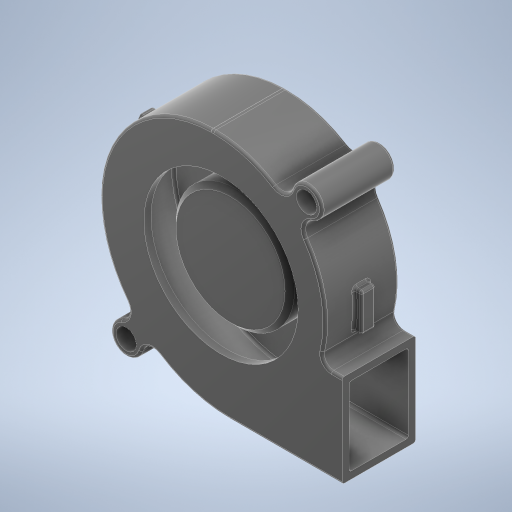
# Autodesk Inventor part: 5015 Fan
Saved by Autodesk Inventor 2024 (Build 280153000, 153)
## iProperties
Created: 2025-01-19
Part Number: 5015 Fan
Material: ABS Plastic
Document SubType Name: Modeling
Designer: Ishaan
Density: 1.06 g/cm^3
Appearance: Smooth - Black
Author: Ishaan
Autodesk Inventor part; units mm, degrees
ref_plane "YZ Plane" through (0, 0, 0) normal (1, 0, 0) x (0, 1, 0)
ref_plane "XZ Plane" through (0, 0, 0) normal (0, 1, 0) x (-1, 0, 0)
ref_plane "XY Plane" through (0, 0, 0) normal (0, 0, 1) x (1, 0, 0)
sketch "Sketch1" plane through (0, 0, 0) normal (0, 0, 1) x (1, 0, 0)
  line L0 (-51.0368, 43.6346) -> (74.9868, 43.6346) construction
  line L1 (74.9868, 43.6346) -> (74.9868, -48.5034) construction
  line L2 (74.9868, -48.5034) -> (-51.0368, -48.5034) construction
  line L3 (-51.0368, -48.5034) -> (-51.0368, 43.6346) construction
  circle A0 centre (0, 0) radius 16.25 construction
  line L4 (0, 0) -> (-20, 0) construction
  line L5 (-20, 0) -> (-20, -23.5) construction
  line L6 (-20, -23.5) -> (0, -23.5) construction
  line L7 (0, -23.5) -> (0, 0) construction
  line L8 (0, 0) -> (18, 0) construction
  line L9 (18, 0) -> (18, 20.5) construction
  line L10 (18, 20.5) -> (0, 20.5) construction
  line L11 (0, 20.5) -> (0, 0) construction
  circle A1 centre (-20, -23.5) radius 2.15 construction
  circle A2 centre (-20, -23.5) radius 3.25
  circle A3 centre (18, 20.5) radius 3.25
  line L12 (25.5, -27.3) -> (-25.5, -27.3)
  line L13 (-25.5, -27.3) -> (-25.5, 23.7)
  line L14 (-25.5, 23.7) -> (25.5, 23.7)
  line L15 (25.5, 23.7) -> (25.5, -27.3)
  line L16 (25.5, -27.3) -> (-25.5, 23.7) construction
  line L17 (-25.5, -27.3) -> (25.5, 23.7) construction
  line L18 (25.5, -7.8) -> (20.5964, -7.8)
  arc A4 (20.5964, -7.8) -> (-1.5, 23.7) centre (-1.5, 0.2) ccw
  arc A5 (-1.5, 23.7) -> (-25.5, 0) centre (-1.7981, 0) ccw
  arc A6 (-25.5, 0) -> (1.8, -27.3) centre (1.8, 0) ccw
  circle A7 centre (12.4829, 22.1198) radius 2.5
  circle A8 centre (19.8402, 15.0524) radius 2.5
  circle A9 centre (-21.8953, -18.0713) radius 2.5
  circle A10 centre (-14.4446, -24.9831) radius 2.5
  line L19 (-51.0368, 43.6346) -> (74.9868, 43.6346) construction
  line L20 (74.9868, 43.6346) -> (74.9868, -48.5034) construction
  line L21 (74.9868, -48.5034) -> (-51.0368, -48.5034) construction
  line L22 (-51.0368, -48.5034) -> (-51.0368, 43.6346) construction
  line L23 (25.5, -27.3) -> (25.5, -7.8)
  point P0 (0, -1.8)
  point P1 (-19.9074, -16.5553)
  point P2 (-21.0713, -20.4316)
  point P3 (-16.86, -24.3383)
  point P4 (-13.0818, -22.8872)
  point P5 (17.7883, 13.6243)
  point P6 (19.0401, 17.4209)
  point P7 (14.8816, 21.4156)
  point P8 (11.1384, 20.0122)
  point P9 (-2.0962, 23.7)
  point P10 (18.5679, 23.7)
  point P11 (17.4321, 23.7)
  point P12 (25.5, -17.55)
  dimension "d1" = 32.5
  dimension "d14" = 20
  dimension "d15" = 23.5
  dimension "d16" = 18
  dimension "d17" = 20.5
  dimension "d38" = 4.3
  dimension "d39" = 6.5
  dimension "d40" = 6.5
  dimension "d41" = 51
  dimension "d42" = 51
  dimension "d44" = 1.8
  dimension "d45" = 19.5
  dimension "d50" = 1.5
  dimension "d56" = 23.5
  dimension "d59" = 5
  dimension "d100" = 17.55
  constraints: 32 end point, 12 tangent, 11 centre point, 6 coincident, 6 parallel, 6 point on circle, 5 horizontal, 5 point on line, 4 perpendicular, 4 vertical, 3 equal radius, 3 midpoint, 1 horizontal alignment, 4 other
  measures "d1" diameter of A0
  measures "d14" distance of L6.end L5.end
  measures "d15" distance of L5.end L4.end
  measures "d16" distance of L10.end L9.end
  measures "d17" distance of L9.end L8.end
  measures "d38" diameter of A1
  measures "d39" diameter of A2
  measures "d40" diameter of A3
  measures "d41" distance of L13.end L14.end
  measures "d42" distance of L12.end L13.end
  measures "d44" distance of point (0, 0) point (0, -1.8)
  measures "d45" distance between parallel lines of L18 L12
  measures "d50" horizontal distance of A4.end point (0, 0)
  measures "d56" radius of A4
  measures "d59" diameter of A8
  measures "d100" vertical distance of point (0, 0) point (25.5, -17.55)
extrude "Extrusion1" add sketch "Sketch1" along normal mid plane 15.5 contours A6 A5 A4 L18 L15 L12
fillet "Fillet1" radius 2 1 edges at (20.5964, -7.8, 0)
shell "Shell1" thickness 1.5 removed faces 1 at (25.5, -14.3, 2.5833)
extrude "Extrusion2" add sketch "Sketch1" along normal up to surface (15.5 mm away) from surface at -7.75 contours A2 | A2 A9 A6 A10 | A7 A3 A8 A4 | A3 L14 | A3 L14
fillet_without_effect "Fillet2"
fillet "Fillet3" radius 0.5 14 edges at (-17.5956, 15.6001, 6.25) (-16.4434, -18.2434, 6.25) (13.65, -25.8, 6.25) (15.7899, 13.8036, 6.25) (20.5334, -7.9642, 6.25) (24.392, -9.3, 6.25) (-1.7981, 22.2, 6.25) (15.7899, 13.8036, -6.25) (-1.7981, 22.2, -6.25) (-17.5956, 15.6001, -6.25) (-16.4434, -18.2434, -6.25) (13.65, -25.8, -6.25) (24.392, -9.3, -6.25) (20.5334, -7.9642, -6.25)
fillet "Fillet4" radius 0.5 24 edges at (-5.9611, -26.1736, 7.75) (-15.3409, -22.6493, 7.75) (-22.2103, -25.8827, 7.75) (-19.5009, -18.7902, 7.75) (-24.0641, -8.7372, 7.75) (-18.663, 16.654, 7.75) (13.65, -27.3, 7.75) (21.7123, -7.0367, 7.75) (21.5979, 4.5286, 7.75) (17.466, 15.8353, 7.75) (20.2514, 22.8438, 7.75) (24.392, -7.8, 7.75) (21.7123, -7.0367, -7.75) (21.5979, 4.5286, -7.75) (17.466, 15.8353, -7.75) (20.2514, 22.8438, -7.75) (24.392, -7.8, -7.75) (-5.9611, -26.1736, -7.75) (-15.3409, -22.6493, -7.75) (-22.2103, -25.8827, -7.75) (-19.5009, -18.7902, -7.75) (-24.0641, -8.7372, -7.75) (-18.663, 16.654, -7.75) (13.65, -27.3, -7.75)
sketch "Sketch2" plane through (0, 0, 7.75) normal (0, 0, 1) x (1, 0, 0)
  circle A0 centre (0, 0) radius 16.25 projected
extrude "Extrusion3" cut sketch "Sketch2" against normal up to surface (14 mm away)
sketch "Sketch3" plane through (1.8, -25.3, -6.25) normal (0, 0, 1) x (1, 0, 0)
  circle A0 centre (-1.8, 25.3) radius 12.5
  point P0 (-1.8, 25.3)
  dimension "d71" = 25
  constraints: 1 centre point, 1 coincident
  measures "d71" diameter of A0
extrude "Extrusion4" add sketch "Sketch3" along normal blind 12
chamfer "Chamfer1" distance 1 angle 45 1 edges at (-12.5, 0, 5.75)
sketch "Sketch4" plane through (0, 0, 7.75) normal (0, 0, 1) x (1, 0, 0)
  circle A0 centre (0, 0) radius 16.25 projected
  line L0 (23.2841, -8.3) -> (25.5, -8.3) projected
  arc A1 (20.8543, -5.2118) -> (23.2841, -8.3) centre (23.2841, -5.8) ccw projected
  arc A2 (20.8543, -5.2118) -> (17.3779, 13.3387) centre (-1.5, 0.2) ccw projected
  arc A3 (18.8801, 17.8946) -> (17.3779, 13.3387) centre (19.8402, 15.0524) ccw projected
  arc A4 (18.8801, 17.8946) -> (15.3614, 21.2747) centre (18, 20.5) ccw projected
  arc A5 (10.8695, 19.5906) -> (15.3614, 21.2747) centre (12.4829, 22.1198) ccw projected
  arc A6 (10.8695, 19.5906) -> (-1.5, 23.2) centre (-1.5, 0.2) ccw projected
  line L1 (-2.0834, 23.2) -> (-1.5, 23.2) projected
  arc A7 (-2.0834, 23.2) -> (-2.1031, 23.1999) centre (-2.0834, 21.7) ccw projected
  arc A8 (-2.1031, 23.1999) -> (-25, 0) centre (-1.7981, 0) ccw projected
  arc A9 (-25, 0) -> (-19.5099, -16.2521) centre (1.8, 0) ccw projected
  arc A10 (-20.9064, -20.9037) -> (-19.5099, -16.2521) centre (-21.8953, -18.0713) ccw projected
  arc A11 (-20.9064, -20.9037) -> (-17.343, -24.2093) centre (-20, -23.5) ccw projected
  arc A12 (-12.8092, -22.468) -> (-17.343, -24.2093) centre (-14.4446, -24.9831) ccw projected
  arc A13 (-12.8092, -22.468) -> (1.8, -26.8) centre (1.8, 0) ccw projected
  line L2 (25.5, -26.8) -> (1.8, -26.8) projected
  line L3 (25.5, -26.8) -> (25.5, -8.3) projected
hole "Hole1" at (-20, -23.5, 7.75) at (18, 20.5, 7.75) direction (0, 0, -1) diameter 4.3 end through all
sketch "Sketch5" plane through (0, 0, 0) normal (0, 0, 1) x (1, 0, 0)
  circle A0 centre (0, 0) radius 12.5 projected
  arc A1 (-24, 0) -> (1.8, -25.8) centre (1.8, 0) ccw projected
  line L0 (1.8, -25.8) -> (25.5, -25.8) projected
  line L1 (25.5, -25.8) -> (25.5, -27.3) projected
  line L2 (25.5, -27.3) -> (1.8, -27.3) projected
  arc A2 (-2.1006, 22.1998) -> (-24, 0) centre (-1.7981, 0) ccw projected
  arc A3 (-2.0734, 22.2) -> (-2.1006, 22.1998) centre (-2.0734, 20.2) ccw projected
  line L3 (-1.5, 22.2) -> (-2.0734, 22.2) projected
  arc A4 (19.8823, -4.9765) -> (-1.5, 22.2) centre (-1.5, 0.2) ccw projected
  arc A5 (19.8823, -4.9765) -> (23.2841, -9.3) centre (23.2841, -5.8) ccw projected
  line L4 (25.5, -9.3) -> (23.2841, -9.3) projected
  line L5 (25.5, -7.8) -> (25.5, -9.3) projected
  line L6 (23.2841, -7.8) -> (25.5, -7.8) projected
  arc A6 (21.3402, -5.3294) -> (23.2841, -7.8) centre (23.2841, -5.8) ccw projected
  line L7 (-2.0834, 23.7) -> (-1.5, 23.7) projected
  arc A7 (-2.0834, 23.7) -> (-2.1097, 23.6998) centre (-2.0834, 21.7) ccw projected
  arc A8 (-2.1097, 23.6998) -> (-25.5, 0) centre (-1.7981, 0) ccw projected
  line L8 (22.55, -27.3) -> (14.55, -27.3)
  line L9 (14.55, -27.3) -> (14.55, -28.55)
  line L10 (14.55, -28.55) -> (22.55, -28.55)
  line L11 (22.55, -28.55) -> (22.55, -27.3)
  line L12 (-25.0005, 4.8405) -> (-22.0685, 12.2838)
  line L13 (-22.0685, 12.2838) -> (-23.4641, 12.8336)
  line L14 (-23.4641, 12.8336) -> (-26.3961, 5.3903)
  line L15 (-26.3961, 5.3903) -> (-25.0005, 4.8405)
  line L16 (0, 0) -> (-20, 0) construction
  arc A9 (21.3402, -5.3294) -> (-1.5, 23.7) centre (-1.5, 0.2) ccw projected
  line L17 (21.5454, -4.4) -> (21.5454, 3.6)
  line L18 (21.5454, 3.6) -> (23.3454, 3.6)
  line L19 (23.3454, 3.6) -> (23.3454, -4.4)
  line L20 (23.3454, -4.4) -> (21.5454, -4.4)
  circle A10 centre (18, 20.5) radius 2.15 projected
  circle A11 centre (-20, -23.5) radius 2.15 projected
  arc A12 (-13.0818, -22.8872) -> (1.8, -27.3) centre (1.8, 0) ccw projected
  arc A13 (-13.0818, -22.8872) -> (-16.86, -24.3383) centre (-14.4446, -24.9831) ccw projected
  arc A14 (-21.0713, -20.4316) -> (-16.86, -24.3383) centre (-20, -23.5) ccw projected
  arc A15 (-21.0713, -20.4316) -> (-19.9074, -16.5553) centre (-21.8953, -18.0713) ccw projected
  arc A16 (-25.5, 0) -> (-19.9074, -16.5553) centre (1.8, 0) ccw projected
  arc A17 (11.1384, 20.0122) -> (-1.5, 23.7) centre (-1.5, 0.2) ccw projected
  arc A18 (11.1384, 20.0122) -> (14.8816, 21.4156) centre (12.4829, 22.1198) ccw projected
  arc A19 (19.0401, 17.4209) -> (14.8816, 21.4156) centre (18, 20.5) ccw projected
  arc A20 (19.0401, 17.4209) -> (17.7883, 13.6243) centre (19.8402, 15.0524) ccw projected
  arc A21 (21.3402, -5.3294) -> (17.7883, 13.6243) centre (-1.5, 0.2) ccw projected
  point P0 (18.55, -28.55)
  point P1 (21.5454, -0.4)
  dimension "d88" = 8
  dimension "d89" = 6.95
  dimension "d90" = 1.25
  dimension "d91" = 8
  dimension "d92" = 1.5
  dimension "d93" = 21.5
  dimension "d94" = 1.8
  dimension "d95" = 8
  dimension "d96" = 0.4
  constraints: 24 end point, 6 parallel, 3 perpendicular, 3 point on circle, 2 midpoint, 1 horizontal, 1 point on line, 1 vertical
  measures "d88" distance of L10.end L9.end
  measures "d89" distance from line of point (18.55, -28.55) L1
  measures "d90" distance between parallel lines of L2 L10
  measures "d91" distance of L13.end L14.end
  measures "d92" distance of L12.end L13.end
  measures "d93" angle of L15 L16
  measures "d94" distance of L17.end L18.end
  measures "d95" distance of L18.end L19.end
  measures "d96" vertical distance of point (0, 0) point (21.545, -0.4)
extrude "Extrusion5" add sketch "Sketch5" along normal mid plane 3 contours L11 L10 L9 L2 | L17 L18 A9 | A9 L18 L19 L20 | L15 L14 L13 A8 | A8 L12
fillet "Fillet5" radius 0.5 36 edges at (18.55, -27.3, 1.5) (22.55, -27.3, 0) (14.55, -27.3, 0) (18.55, -27.3, -1.5) (22.55, -27.925, 1.5) (14.55, -27.925, 1.5) (14.55, -28.55, 0) (18.55, -28.55, 1.5) (22.55, -28.55, 0) (14.55, -27.925, -1.5) (18.55, -28.55, -1.5) (22.55, -27.925, -1.5) (22.4454, -4.4, -1.5) (21.5454, -4.4, 0) (22.4454, -4.4, 1.5) (21.9921, -0.4089, -1.5) (23.3454, -4.4, 0) (23.3454, -0.4, -1.5) (22.5491, 3.6, -1.5) (23.3454, -0.4, 1.5) (23.3454, 3.6, 0) (21.9921, -0.4089, 1.5) (22.5491, 3.6, 1.5) (21.7527, 3.6, 0) (-22.0685, 12.2838, 0) (-22.7663, 12.5587, -1.5) (-22.7663, 12.5587, 1.5) (-23.4641, 12.8336, 0) (-23.8508, 8.6868, -1.5) (-23.8508, 8.6868, 1.5) (-25.6983, 5.1154, -1.5) (-25.6983, 5.1154, 1.5) (-25.0005, 4.8405, 0) (-24.9301, 9.1119, -1.5) (-26.3961, 5.3903, 0) (-24.9301, 9.1119, 1.5)
body "Solid1"
